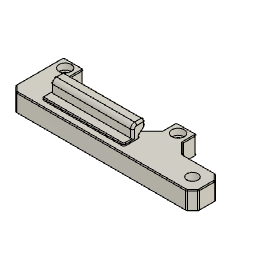
RS25 Vertical Mount (Autodesk Fusion 360 design; units mm, degrees)
Autodesk Fusion 360 part; units mm, degrees
sketch "Sketch1" plane through (0, 0, 0) normal (0, 0, 1) x (1, 0, 0)
  line L0 (32.5, 13.1) -> (-32.5, 13.1)
  line L1 (-32.5, 13.1) -> (-32.5, -13.1)
  line L2 (-32.5, -13.1) -> (32.5, -13.1)
  line L3 (32.5, -13.1) -> (32.5, 13.1)
  line L4 (32.5, 13.1) -> (-32.5, -13.1) construction
  line L5 (-32.5, 13.1) -> (32.5, -13.1) construction
  line L6 (32.5, -13.1) -> (56.5, -13.1)
  line L7 (56.5, -13.1) -> (56.5, 1.1)
  line L8 (56.5, 1.1) -> (32.5, 1.1)
  dimension "d1" = 65
  dimension "d2" = 26.2
  dimension "d4" = 14.2
  dimension "d79" = 24
  constraint horizontal L0
  constraint perpendicular L0 L1
  constraint parallel L0 L2
  constraint parallel L1 L3
  constraint coincident L4 origin
  constraint coincident L5 origin
  constraint perpendicular L3 L6
  constraint perpendicular L6 L7
  constraint coincident L3 L8.end
  constraint perpendicular L3 L8
  measures "d1" distance of L1.end L2.end
  measures "d2" distance of L0.end L1.end
  measures "d4" distance of L6.end L7.end
  measures "d79" distance of L2.end L6.end
extrude "Extrude1" add sketch "Sketch1" along normal blind 9
sketch "Sketch2" plane through (0, 0, 9) normal (0, 0, 1) x (-1, 0, 0)
  line L0 (-56.5, -1.1) -> (-32.5, -1.1)
  line L1 (-32.5, -1.1) -> (-32.5, -13.1)
  line L2 (-32.5, -13.1) -> (32.5, -13.1)
  line L3 (32.5, -13.1) -> (32.5, 13.1)
  line L4 (32.5, 13.1) -> (-56.5, 13.1)
  line L5 (-56.5, 13.1) -> (-56.5, -1.1)
  line L6 (27.5, -8.9) -> (-27.5, -8.9) construction
  line L7 (0, -8.9) -> (0, -13.1) construction
  dimension "d7" = 55
  dimension "d8" = 4.2
  constraint parallel L2 L6
  constraint midpoint L6 L7.start
  constraint perpendicular L2 L7
  constraint midpoint L2 L7.end
  measures "d7" distance of L6.start L6.end
  measures "d8" distance of L7.start L7.end
hole "Hole1" at (-27.5, 8.9, 9) at (27.5, 8.9, 9) direction (0, 0, -1) diameter 3.4 end through all counterbore diameter 6 counterbore depth 3
sketch "Sketch4" plane through (0, 0, 0) normal (0, 0, -1) x (1, 0, 0)
  circle A0 centre (-27.5, -8.9) radius 1.7
  circle A1 centre (27.5, -8.9) radius 1.7
  line L0 (32.5, -1.1) -> (56.5, -1.1)
  line L1 (56.5, -1.1) -> (56.5, 13.1)
  line L2 (56.5, 13.1) -> (-32.5, 13.1)
  line L3 (-32.5, 13.1) -> (-32.5, -13.1)
  line L4 (-32.5, -13.1) -> (32.5, -13.1)
  line L5 (32.5, -13.1) -> (32.5, -1.1)
  line L6 (56.5, 6) -> (49.4, 6) construction
  dimension "d27" = 7.1
  constraint midpoint L1 L6.start
  constraint perpendicular L1 L6
  measures "d27" distance of L6.start L6.end
hole "Hole2" at (49.4, -6, 0) direction (0, 0, 1) diameter 5.4 depth 9 tip angle 118 counterbore diameter 9.8 counterbore depth 3
sketch "Sketch5" plane through (0, 0, 9) normal (0, 0, 1) x (-1, 0, 0)
  circle A0 centre (-49.4, 6) radius 2.7
  circle A1 centre (27.5, -8.9) radius 3
  circle A2 centre (-27.5, -8.9) radius 3
  line L0 (-56.5, -1.1) -> (-32.5, -1.1)
  line L1 (-32.5, -1.1) -> (-32.5, -13.1)
  line L2 (-32.5, -13.1) -> (32.5, -13.1)
  line L3 (32.5, -13.1) -> (32.5, 13.1)
  line L4 (32.5, 13.1) -> (-56.5, 13.1)
  line L5 (-56.5, 13.1) -> (-56.5, -1.1)
  line L6 (20, 2) -> (-20, 2)
  line L7 (-20, 2) -> (-20, 5.8)
  line L8 (-20, 5.8) -> (20, 5.8)
  line L9 (20, 5.8) -> (20, 2)
  line L10 (0, 2) -> (0, -13.1) construction
  dimension "d23" = 7.3
  dimension "d25" = 3.8
  dimension "d26" = 40
  constraint horizontal L6
  constraint vertical L7
  constraint horizontal L8
  constraint vertical L9
  constraint midpoint L6 L10.start
  constraint perpendicular L6 L10
  constraint midpoint L2 L10.end
  measures "d23" distance of L4 L8
  measures "d25" distance of L6.start L8.end
  measures "d26" distance of L6.start L6.end
extrude "Extrude2" add sketch "Sketch5" along normal blind 6.8 contours L6 L7 L8 L9
sketch "Sketch6" plane through (0, 0, 9) normal (0, 0, 1) x (-1, 0, 0)
  line L0 (20, 5.8) -> (20, 2)
  line L1 (20, 2) -> (-20, 2)
  line L2 (-20, 2) -> (-20, 5.8)
  line L3 (-20, 5.8) -> (20, 5.8)
  circle A0 centre (-49.4, 6) radius 2.7
  circle A1 centre (27.5, -8.9) radius 3
  circle A2 centre (-27.5, -8.9) radius 3
  line L4 (-56.5, -1.1) -> (-32.5, -1.1)
  line L5 (-32.5, -1.1) -> (-32.5, -13.1)
  line L6 (-32.5, -13.1) -> (32.5, -13.1)
  line L7 (32.5, -13.1) -> (32.5, 13.1)
  line L8 (32.5, 13.1) -> (-56.5, 13.1)
  line L9 (-56.5, 13.1) -> (-56.5, -1.1)
  line L10 (20, 5.8) -> (20, 10)
  line L11 (20, 10) -> (-20, 10)
  line L12 (-20, 10) -> (-20, 5.8)
  dimension "d30" = 4.2
  constraint coincident L0.start L3.end
  constraint perpendicular L3 L10
  constraint perpendicular L2 L11
  constraint coincident L2.end L3.start
  constraint perpendicular L3 L12
  measures "d30" distance of L11.end L2.end
extrude "Extrude3" add sketch "Sketch6" along normal blind 1 contours L3 L10 L11 L12
sketch "Sketch7" plane through (20, 0, 0) normal (1, 0, 0) x (0, 1, 0)
  line L0 (-10, 9) -> (-2, 9)
  line L1 (-2, 9) -> (-2, 15.8)
  line L2 (-2, 15.8) -> (-5.8, 15.8)
  line L3 (-5.8, 15.8) -> (-5.8, 10)
  line L4 (-5.8, 10) -> (-10, 10)
  line L5 (-10, 10) -> (-10, 9)
  line L6 (-2, 15.8) -> (0.5, 15.8)
  line L7 (0.5, 15.8) -> (0.5, 13.2977)
  line L8 (0.5, 13.2977) -> (-2, 11.2)
  dimension "d33" = 6.3
  dimension "d34" = 130
  dimension "d35" = 2.2
  constraint coincident L1.end L2.start
  constraint perpendicular L1 L6
  constraint perpendicular L6 L7
  constraint coincident L1 L8.end
  measures "d33" distance of L2.end L6.end
  measures "d34" angle of L1 L8
  measures "d35" distance of L0.end L8.end
extrude "Extrude4" add sketch "Sketch7" against normal up to surface (40 mm away) contours L1 L6 L7 L8
sketch "Sketch9" plane through (0, 0, 9) normal (0, 0, 1) x (-1, 0, 0)
  line L0 (20, 10) -> (20, 2)
  line L1 (20, 2) -> (-20, 2)
  line L2 (-20, 2) -> (-20, 10)
  line L3 (-20, 10) -> (20, 10)
  circle A0 centre (-49.4, 6) radius 2.7
  circle A1 centre (27.5, -8.9) radius 3
  circle A2 centre (-27.5, -8.9) radius 3
  line L4 (-56.5, -1.1) -> (-32.5, -1.1)
  line L5 (-32.5, -1.1) -> (-32.5, -13.1)
  line L6 (-32.5, -13.1) -> (32.5, -13.1)
  line L7 (32.5, -13.1) -> (32.5, 13.1)
  line L8 (32.5, 13.1) -> (-56.5, 13.1)
  line L9 (-56.5, 13.1) -> (-56.5, -1.1)
  line L10 (22.5, -13.1) -> (22.5, -1.1)
  line L11 (22.5, -1.1) -> (-22.5, -1.1)
  line L12 (-22.5, -1.1) -> (-22.5, -13.1)
  line L13 (0, -1.1) -> (0, -13.1) construction
  dimension "d57" = 90
  dimension "d59" = 10
  constraint coincident L6 L10.start
  constraint parallel L6 L11
  constraint coincident L6 L12.end
  constraint midpoint L11 L13.start
  constraint perpendicular L11 L13
  constraint midpoint L6 L13.end
  constraint symmetric L10 L12 L13
  constraint collinear L4 L11
  measures "d57" angle of L6 L10
  measures "d59" distance of L5.end L12.end
extrude "Extrude6" cut sketch "Sketch9" against normal through all contours L6 L10 L11 L12
sketch "Sketch10" plane through (0, 0, 3) normal (0, 0, -1) x (1, 0, 0)
  circle A0 centre (49.4, 6) radius 4.9
  circle A1 centre (49.4, 6) radius 2.7
  line L0 (45.311, 8.7) -> (53.489, 8.7)
  line L1 (45.311, 3.3) -> (53.489, 3.3)
  constraint coincident A0 L0.start
  constraint coincident A0 L0.end
  constraint horizontal L0
  constraint coincident A0 L1.start
  constraint coincident A0 L1.end
  constraint parallel L0 L1
  constraint tangent A1 L1
  constraint tangent A1 L0
extrude "Extrude7" add sketch "Sketch10" along normal blind 0.2 contours A0 L0 | A0 L1
sketch "Sketch11" plane through (0, 0, 3) normal (0, 0, -1) x (1, 0, 0)
  line L0 (53.489, 8.7) -> (49.4, 8.7)
  arc A0 (49.4, 3.3) -> (49.4, 8.7) centre (49.4, 6) ccw
  line L1 (49.4, 3.3) -> (53.489, 3.3)
  arc A1 (53.489, 3.3) -> (53.489, 8.7) centre (49.4, 6) ccw
  line L2 (49.4, 8.7) -> (45.311, 8.7)
  arc A2 (45.311, 8.7) -> (45.311, 3.3) centre (49.4, 6) ccw
  line L3 (45.311, 3.3) -> (49.4, 3.3)
  arc A3 (49.4, 8.7) -> (49.4, 3.3) centre (49.4, 6) ccw
  line L4 (52.1, 8.7) -> (52.1, 3.3)
  line L5 (46.7, 8.7) -> (46.7, 3.3)
  constraint coincident L0 L4.start
  constraint coincident L1 L4.end
  constraint perpendicular L1 L4
  constraint coincident L2 L5.start
  constraint coincident L3 L5.end
  constraint perpendicular L3 L5
  constraint tangent A3 L5
  constraint tangent A0 L4
extrude "Extrude8" cut sketch "Sketch11" against normal blind 0.2 contours L0 A0 L4 | L2 A3 L5 | A0 L1 L4 | L3 A3 L5
chamfer "Chamfer5" distance 5 angle 45 3 edges at (22.5, 1.1, 4.5) (-22.5, 1.1, 4.5) (32.5, 1.1, 4.5)
chamfer "Chamfer2" distance 3 angle 45 3 edges at (56.5, 1.1, 4.5) (-32.5, -13.1, 4.5) (56.5, -13.1, 4.5)
sketch "Sketch13" plane through (0, 0, 0) normal (0, 0, -1) x (1, 0, 0)
  line L0 (56.5, 10.1) -> (53.5, 13.1)
  line L1 (53.5, 13.1) -> (-29.5, 13.1)
  line L2 (-29.5, 13.1) -> (-32.5, 10.1)
  line L3 (-32.5, 10.1) -> (-32.5, -13.1)
  line L4 (-32.5, -13.1) -> (-22.5, -13.1)
  line L5 (-22.5, -13.1) -> (-22.5, -6.1)
  line L6 (-22.5, -6.1) -> (-17.5, -1.1)
  line L7 (-17.5, -1.1) -> (17.5, -1.1)
  line L8 (17.5, -1.1) -> (22.5, -6.1)
  line L9 (22.5, -6.1) -> (22.5, -13.1)
  line L10 (22.5, -13.1) -> (32.5, -13.1)
  line L11 (32.5, -13.1) -> (32.5, -6.1)
  line L12 (32.5, -6.1) -> (37.5, -1.1)
  line L13 (37.5, -1.1) -> (53.5, -1.1)
  line L14 (53.5, -1.1) -> (56.5, 1.9)
  line L15 (56.5, 1.9) -> (56.5, 10.1)
  circle A0 centre (49.4, 6) radius 4.9
  circle A1 centre (-27.5, -8.9) radius 1.7
  circle A2 centre (27.5, -8.9) radius 1.7
  line L16 (39.5, 3.3) -> (-26.5, 3.3)
  line L17 (-26.5, 3.3) -> (-26.5, 8.7)
  line L18 (-26.5, 8.7) -> (39.5, 8.7)
  line L19 (39.5, 8.7) -> (39.5, 3.3)
  dimension "d72" = 4.4
  dimension "d73" = 4.4
  dimension "d74" = 6
  dimension "d75" = 66
  constraint horizontal L16
  constraint vertical L17
  constraint horizontal L18
  constraint vertical L19
  measures "d72" distance of L1 L18
  measures "d73" distance of L7 L16
  measures "d74" distance of L3 L17
  measures "d75" distance of L17.end L18.end
extrude "Extrude9" cut sketch "Sketch13" against normal blind 2.8 contours L16 L17 L18 L19
fillet "Fillet1" radius 1 20 edges at (-32.5, 13.1, 4.5) (-32.5, -10.1, 4.5) (-29.5, -13.1, 4.5) (56.5, -1.9, 4.5) (53.5, 1.1, 4.5) (32.5, 13.1, 4.5) (22.5, 13.1, 4.5) (-22.5, 13.1, 4.5) (22.5, 6.1, 4.5) (17.5, 1.1, 4.5) (-17.5, 1.1, 4.5) (-22.5, 6.1, 4.5) (56.5, -10.1, 4.5) (53.5, -13.1, 4.5) (37.5, 1.1, 4.5) (32.5, 6.1, 4.5) (39.5, -3.3, 1.4) (39.5, -8.7, 1.4) (-26.5, -3.3, 1.4) (-26.5, -8.7, 1.4)
fillet "Fillet2" radius 2 1 edges at (0, -5.8, 15.8)
fillet "Fillet3" radius 1 13 edges at (20, -2, 10.1) (-20, -2, 10.1) (20, 0.5, 14.5489) (-20, 0.5, 14.5489) (20, -5.8, 11.9) (20, -5.2142, 15.2142) (20, -1.65, 15.8) (-20, -1.65, 15.8) (-20, -5.2142, 15.2142) (-20, -5.8, 11.9) (0, 0.5, 15.8) (20, -10, 9.5) (-20, -10, 9.5)
chamfer "Chamfer4" distance 0.4 angle 45 37 edges at (19.7071, -9.7071, 10) (20, -6.9, 10) (-20, -6.9, 10) (-19.7071, -9.7071, 10) (0, -10, 10) (37.5315, 1.1761, 9) (45.5, 1.1, 9) (53.4685, 1.0239, 9) (55, -0.4, 9) (56.4239, -1.9315, 9) (56.5, -6, 9) (56.4239, -10.0685, 9) (55, -11.6, 9) (53.4685, -13.0239, 9) (12, -13.1, 9) (-29.4685, -13.0239, 9) (-31, -11.6, 9) (-32.4239, -10.0685, 9) (-32.5, 1.2071, 9) (-32.2071, 12.8071, 9) (-27.5, 13.1, 9) (-22.7929, 12.8071, 9) (-22.5, 9.3071, 9) (-22.4239, 6.1315, 9) (-20, 3.6, 9) (-17.4685, 1.1761, 9) (0, 1.1, 9) (17.4685, 1.1761, 9) (20, 3.6, 9) (22.4239, 6.1315, 9) (22.5, 9.3071, 9) (22.7929, 12.8071, 9) (27.5, 13.1, 9) (32.2071, 12.8071, 9) (32.5, 9.3071, 9) (32.5761, 6.1315, 9) (35, 3.6, 9) 1 faces at (26.1667, 1.3, 0)
equation "d8 = 3 mm + 1.2 mm"
equation "beam_size = 3 mm"
